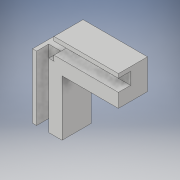
# Autodesk Inventor part: BalsaJig
Saved by Autodesk Inventor 2018 (Build 220112000, 112)
## iProperties
Created: 2018-12-01
Part Number: BalsaJig
Material: Generic
Document SubType Name: Modeling
Designer: F8PLTW
Density: 1 g/cm^3
Appearance: Default
Author: F8PLTW
Autodesk Inventor part; units mm, degrees
ref_plane "YZ Plane" through (0, 0, 0) normal (1, 0, 0) x (0, 1, 0)
ref_plane "XZ Plane" through (0, 0, 0) normal (0, 1, 0) x (-1, 0, 0)
ref_plane "XY Plane" through (0, 0, 0) normal (0, 0, 1) x (1, 0, 0)
sketch "Sketch1" plane through (0, 0, 0) normal (0, 0, 1) x (1, 0, 0)
  line L0 (-30.4239, 15.0503) -> (-5.0239, 15.0503)
  line L1 (-5.0239, 15.0503) -> (-5.0239, -10.3497)
  line L2 (-5.0239, -10.3497) -> (-30.4239, -10.3497)
  line L3 (-30.4239, -10.3497) -> (-30.4239, 15.0503)
  point P0 (0, 0)
  dimension "d0" = 25.4
  dimension "d1" = 25.4
  constraints: 8 end point, 2 parallel, 1 horizontal, 1 perpendicular
  measures "d0" distance of L1.end L2.end
  measures "d1" distance of L0.end L1.end
extrude "Extrusion1" add sketch "Sketch1" along normal blind 6.6
sketch "Sketch2" plane through (0, 0, 6.6) normal (0, 0, 1) x (1, 0, 0)
  line L0 (-5.0239, 15.0503) -> (-30.4239, 15.0503) projected
  line L1 (-30.4239, 15.0503) -> (-24.0739, 15.0503)
  line L2 (-24.0739, 15.0503) -> (-24.0739, 8.7003)
  line L3 (-24.0739, 8.7003) -> (-30.4239, 8.7003)
  line L4 (-30.4239, 8.7003) -> (-30.4239, 15.0503)
  point P0 (0, 0)
  dimension "d4" = 6.35
  dimension "d5" = 6.35
  constraints: 8 end point, 2 parallel, 1 horizontal, 1 perpendicular
  measures "d4" distance of L2.end L3.end
  measures "d5" distance of L1.end L2.end
extrude "Extrusion2" cut sketch "Sketch2" against normal blind 6.6
sketch "Sketch3" plane through (0, 0, 6.6) normal (0, 0, 1) x (1, 0, 0)
  line L0 (-5.0239, 15.0503) -> (-24.0739, 15.0503) projected
  line L1 (-24.0739, 8.7003) -> (-24.0739, 15.0503) construction
  line L2 (-24.0739, 15.0503) -> (-24.0739, 8.7003) construction
  line L3 (-30.4239, 8.7003) -> (-24.0739, 8.7003) construction
  line L4 (-24.0739, 8.7003) -> (-30.4239, 8.7003) construction
  line L5 (-27.2489, 8.7003) -> (-27.2489, -10.3839) construction
  line L6 (-24.0739, 11.8753) -> (-5.0239, 11.8753) construction
  line L7 (-5.0239, -10.3497) -> (-5.0239, 15.0503) projected
  line L8 (-5.0239, 13.5009) -> (-5.0239, 10.2497)
  line L9 (-5.0239, 10.2497) -> (-24.0739, 10.2497)
  line L10 (-24.0739, 10.2497) -> (-24.0739, 13.5009)
  line L11 (-30.4239, -10.3497) -> (-5.0239, -10.3497) projected
  line L12 (-28.8745, 8.7003) -> (-25.6233, 8.7003)
  line L13 (-25.6233, 8.7003) -> (-25.6233, -10.3497)
  line L14 (-25.6233, -10.3497) -> (-28.8745, -10.3497)
  line L15 (-28.8745, -10.3497) -> (-29.2301, -10.3497)
  line L16 (-29.2301, -10.3497) -> (-29.2301, 8.7003)
  line L17 (-28.8745, 8.7003) -> (-29.2301, 8.7003)
  line L18 (-24.0739, 13.5009) -> (-24.0739, 13.8565)
  line L19 (-24.0739, 13.8565) -> (-5.0239, 13.8565)
  line L20 (-5.0239, 13.8565) -> (-5.0239, 13.5009)
  point P0 (0, 0)
  dimension "d8" = 3.2512
  dimension "d20" = 0.3556
  dimension "d21" = 0.3556
  constraints: 32 end point, 9 point on line, 5 perpendicular, 4 equal length, 2 horizontal, 2 midpoint, 1 vertical
  measures "d8" distance of L8.start L8.end
  measures "d20" distance of L14.end L15.end
  measures "d21" distance of L10.end L18.end
extrude "Extrusion3" cut sketch "Sketch3" against normal blind 1.6
sketch "Sketch4" plane through (0, 0, 6.6) normal (0, 0, 1) x (1, 0, 0)
  line L0 (-24.0739, 8.7003) -> (-25.6233, 8.7003) projected
  line L1 (-25.6233, 8.7003) -> (-24.0739, 8.7003)
  line L2 (-5.0239, 10.2497) -> (-24.0739, 10.2497) projected
  line L3 (-24.0739, 8.7003) -> (-24.0739, 10.2497)
  line L4 (-24.0739, 10.2497) -> (-5.0239, 10.2497)
  line L5 (-5.0239, -10.3497) -> (-5.0239, 10.2497) projected
  line L6 (-5.0239, 10.2497) -> (-5.0239, -10.3497)
  line L7 (-5.0239, -10.3497) -> (-25.6233, -10.3497)
  line L8 (-5.0239, -10.3497) -> (-30.4239, -10.3497) projected
  line L9 (-25.6233, 8.7003) -> (-25.6233, -10.3497)
  point P0 (0, 0)
  constraints: 12 end point, 3 collinear, 2 perpendicular, 1 point on line
extrude "Extrusion4" add sketch "Sketch4" along normal blind 2
sketch "Sketch5" plane through (0, 0, 6.6) normal (0, 0, 1) x (1, 0, 0)
  line L0 (-5.0239, 15.0503) -> (-24.0739, 15.0503) projected
  line L1 (-24.0739, 15.0503) -> (-5.0239, 15.0503)
  line L2 (-30.4239, -10.3497) -> (-30.4239, 8.7003)
  line L3 (-30.4239, 8.7003) -> (-29.2301, 8.7003)
  line L4 (-30.4239, 8.7003) -> (-24.0739, 8.7003) projected
  line L5 (-29.2301, 8.7003) -> (-29.2301, -10.3497)
  line L6 (-30.4239, -10.3497) -> (-29.2301, -10.3497) projected
  line L7 (-29.2301, -10.3497) -> (-30.4239, -10.3497)
  line L8 (-24.0739, 15.0503) -> (-24.0739, 13.8565) projected
  line L9 (-24.0739, 15.0503) -> (-24.0739, 13.8565)
  line L10 (-24.0739, 13.8565) -> (-5.0239, 13.8565)
  line L11 (-5.0239, 13.8565) -> (-5.0239, 15.0503) projected
  point P0 (0, 0)
  point P1 (-5.0239, 13.5009)
  point P2 (-28.8745, -10.3497)
  point P3 (-24.0739, 13.5009)
  dimension "d18" = 1.1938
  dimension "d19" = 1.1938
  constraints: 16 end point, 3 perpendicular, 1 horizontal, 1 point on line
  measures "d18" distance of L2.end L3.end
  measures "d19" distance of L0.end L8.end
extrude "Extrusion5" add sketch "Sketch5" along normal blind 2
sketch "Sketch6" plane through (0, 0, 8.6) normal (0, 0, 1) x (1, 0, 0)
  line L0 (-25.6233, -10.3497) -> (-5.0239, -10.3497) projected
  line L1 (-5.0239, -10.3497) -> (-21.6937, -10.3497)
  line L2 (-21.6937, -10.3497) -> (-21.6937, 6.1438)
  line L3 (-21.6937, 6.1438) -> (-5.0239, 6.1438)
  line L4 (-5.0239, 6.1438) -> (-5.0239, -10.3497)
  point P0 (0, 0)
  constraints: 8 end point, 2 parallel, 1 horizontal, 1 perpendicular
extrude "Extrusion6" cut sketch "Sketch6" against normal blind 9
body "Solid1"
